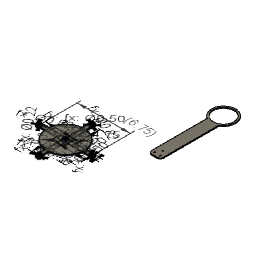
Rocket Platform v8 (Autodesk Fusion 360 design; units mm, degrees)
Autodesk Fusion 360 part; units mm, degrees
note: some values were not read from the file. Set by a fixed rule: which sketch regions a step uses.
sketch "Sketch2" plane through (0, 0, 0) normal (0, 1, 0) x (1, 0, 0)
  circle A0 centre (0, 0) radius 60.325
  circle A1 centre (0, 85.725) radius 6.35
  line L0 (6.35, 0) -> (-6.35, 0)
  line L1 (-6.35, 0) -> (-6.35, 85.725)
  line L2 (-6.35, 85.725) -> (6.35, 85.725)
  line L3 (6.35, 85.725) -> (6.35, 0)
  line L4 (85.725, -6.35) -> (0, -6.35)
  line L5 (0, -6.35) -> (0, 6.35)
  line L6 (0, 6.35) -> (85.725, 6.35)
  line L7 (85.725, 6.35) -> (85.725, -6.35)
  line L8 (-6.35, 0) -> (6.35, 0)
  line L9 (6.35, 0) -> (6.35, -85.725)
  line L10 (6.35, -85.725) -> (-6.35, -85.725)
  line L11 (-6.35, -85.725) -> (-6.35, 0)
  line L12 (0, 6.35) -> (-85.725, 6.35)
  line L13 (-85.725, 6.35) -> (-85.725, -6.35)
  line L14 (-85.725, -6.35) -> (0, -6.35)
  line L15 (0, -6.35) -> (0, 6.35)
  circle A2 centre (-85.725, 0) radius 6.35
  circle A3 centre (0, -85.725) radius 6.35
  circle A4 centre (85.725, 0) radius 6.35
  circle A5 centre (-85.725, 0) radius 2.8
  circle A6 centre (85.725, 0) radius 2.8
  circle A7 centre (0, 85.725) radius 2.8
  circle A8 centre (0, -85.725) radius 2.8
  dimension "d6" = 120.65
  dimension "d7" = 12.7
  dimension "d9" = 12.7
  dimension "d10" = 85.725
  dimension "d11" = 85.725
  dimension "d12" = 12.7
  dimension "d13" = 12.7
  dimension "d14" = 85.725
  dimension "d15" = 85.725
  dimension "d16" = 12.7
  dimension "d17" = 12.7
  dimension "d18" = 12.7
  dimension "d19" = 12.7
  dimension "d24" = 5.6
  dimension "d25" = 5.6
  dimension "d26" = 5.6
  dimension "d27" = 5.6
  dimension "d28" = 171.45
  constraint coincident A0.centre origin
  constraint horizontal L0
  constraint vertical L1
  constraint horizontal L2
  constraint vertical L3
  constraint midpoint A0.centre L0
  constraint midpoint A1.centre L2
  constraint horizontal L4
  constraint vertical L5
  constraint horizontal L6
  constraint vertical L7
  constraint midpoint A0.centre L5
  constraint horizontal L8
  constraint vertical L9
  constraint horizontal L10
  constraint vertical L11
  constraint horizontal L12
  constraint vertical L13
  constraint horizontal L14
  constraint vertical L15
  constraint midpoint L13 A2.centre
  constraint midpoint L10 A3.centre
  constraint midpoint L7 A4.centre
  constraint concentric A2 A5
  constraint concentric A4 A6
  constraint concentric A1 A7
  constraint concentric A3 A8
  measures "d6" diameter of A0
  measures "d7" diameter of A1
  measures "d9" distance of L0.start L0.end
  measures "d10" distance of L0.start L2.end
  measures "d11" distance of L4.start L4.end
  measures "d12" distance of L4.start L6.end
  measures "d13" distance of L0.end L0.start
  measures "d14" distance of L0.end L10.end
  measures "d15" distance of L5.end L12.end
  measures "d16" distance of L5.end L4.end
  measures "d17" diameter of A2
  measures "d18" diameter of A3
  measures "d19" diameter of A4
  measures "d24" diameter of A5
  measures "d25" diameter of A6
  measures "d26" diameter of A7
  measures "d27" diameter of A8
  measures "d28" distance of A2.centre A4.centre
extrude "Extrude1" add sketch "Sketch2" along normal blind 3 contours A0 L3 L4 L6 L9 | A0 L4 L6 A4 | A0 L3 L6 | A0 L4 L9 | A0 L1 L3 L6 L12 | A0 A1 L1 L3 | L0 L3 L5 L6 L8 L15 | L7 A4 A6 | L7 A4 A6 | A0 L9 L11 A3 | A0 L4 L9 L11 L14 | L0 L4 L5 L8 L9 L15 | A0 L1 L12 | A1 L2 A7 | A1 L2 A7 | L0 L1 L5 L8 L12 L15 | A0 L11 L14 | L10 A3 A8 | L10 A3 A8 | L0 L5 L8 L11 L14 L15 | A0 L1 L11 L12 L14 | A0 L12 L14 A2 | L13 A2 A5 | L13 A2 A5 makes body 1
sketch "Sketch3" plane through (0, 0, 0) normal (0, 1, 0) x (1, 0, 0)
  circle A0 centre (189.7163, 321.3667) radius 33.5
  circle A1 centre (189.7163, 321.3667) radius 38.5
  line L0 (170.6663, 321.3667) -> (208.7663, 321.3667)
  line L1 (208.7663, 321.3667) -> (208.7663, 107.5267)
  line L2 (198.6063, 97.3667) -> (180.8263, 97.3667)
  line L3 (170.6663, 107.5267) -> (170.6663, 321.3667)
  circle A2 centre (180.8263, 107.5267) radius 2.25
  circle A3 centre (198.6063, 107.5267) radius 2.25
  circle A4 centre (189.7163, 125.3067) radius 2.25
  line L4 (170.6663, 135.4667) -> (208.7663, 135.4667)
  arc A5 (170.6663, 107.5267) -> (180.8263, 97.3667) centre (180.8263, 107.5267) ccw
  arc A6 (198.6063, 97.3667) -> (208.7663, 107.5267) centre (198.6063, 107.5267) ccw
  line L5 (170.6663, 125.3067) -> (208.7663, 125.3067)
  point P0 (208.7663, 97.3667)
  dimension "d31" = 67
  dimension "d32" = 77
  dimension "d34" = 4.5
  dimension "d35" = 4.5
  dimension "d36" = 4.5
  dimension "d37" = 38.1
  dimension "d40" = 10.16
  dimension "d41" = 10.16
  dimension "d42" = 10.16
  dimension "d43" = 10.16
  dimension "d44" = 10.16
  dimension "d45" = 10.16
  dimension "d46" = 185.9
  dimension "d50" = 10.16
  dimension "d52" = 38.1
  constraint concentric A0 A1
  constraint horizontal L0
  constraint vertical L1
  constraint horizontal L2
  constraint vertical L3
  constraint midpoint A0.centre L0
  constraint coincident L3 L4.start
  constraint coincident L1 L4.end
  constraint perpendicular L1 L4
  constraint tangent L2 A5
  constraint tangent L3 A5
  constraint coincident P0 L1
  constraint coincident P0 L2
  constraint tangent L1 A6
  constraint tangent L2 A6
  constraint coincident L3 L5.start
  constraint coincident L1 L5.end
  constraint perpendicular L1 L5
  constraint midpoint A4.centre L5
  measures "d31" diameter of A0
  measures "d32" diameter of A1
  measures "d34" diameter of A2
  measures "d35" diameter of A3
  measures "d36" diameter of A4
  measures "d37" distance of P0 L4.end
  measures "d40" distance of L3 A2.centre
  measures "d41" distance of L2 A2.centre
  measures "d42" distance of L2 A3.centre
  measures "d43" distance of L1 A3.centre
  measures "d44" radius of A5
  measures "d45" radius of A6
  measures "d46" distance of A0.centre L4
  measures "d50" distance of L4 L5
  measures "d52" distance of L1 L3
extrude "Extrude2" add sketch "Sketch3" along normal blind 3 separate body contours A0 A1 L1 L3 | A0 A1 L1 L3 | A1 L1 L3 L4 | L1 L3 A4 L4 L5 | L1 L2 L3 A4 A5 A6 L5 makes body 2
equation "platform_diameter = 4.75 in"
equation "lobe_width = 0.5 in"
equation "d6 = platform_diameter"
equation "d7 = lobe_width"
equation "lobe_length = 1 in"
equation "d9 = lobe_width"
equation "d10 = platform_diameter / 2 + lobe_length"
equation "d11 = platform_diameter / 2 + lobe_length"
equation "d12 = lobe_width"
equation "d13 = lobe_width"
equation "d14 = platform_diameter / 2 + lobe_length"
equation "d15 = platform_diameter / 2 + lobe_length"
equation "d16 = lobe_width"
equation "d17 = lobe_width"
equation "d18 = lobe_width"
equation "d19 = lobe_width"
equation "material_thickness = 3 mm"
equation "d21 = material_thickness"
equation "led_size = 5.6 mm"
equation "d24 = led_size"
equation "d25 = led_size"
equation "d26 = led_size"
equation "d27 = led_size"
equation "upper_hole_diameter = 67 mm"
equation "upper_hole_thickness = 1 cm"
equation "d31 = upper_hole_diameter"
equation "d32 = upper_hole_diameter + upper_hole_thickness"
equation "upper_screw_hole_size = 4.5 mm"
equation "d34 = upper_screw_hole_size"
equation "d35 = upper_screw_hole_size"
equation "d36 = upper_screw_hole_size"
equation "upper_screw_offset = 0.4 in"
equation "d40 = upper_screw_offset"
equation "d41 = upper_screw_offset"
equation "d42 = upper_screw_offset"
equation "d43 = upper_screw_offset"
equation "d44 = upper_screw_offset"
equation "d45 = upper_screw_offset"
equation "d46 = wall_offset + upper_hole_diameter / 2"
equation "wall_offset = 6 in"
equation "d48 = material_thickness"
equation "d50 = upper_screw_offset"
equation "support_bar_width = 1.5 in"
equation "d52 = support_bar_width"
